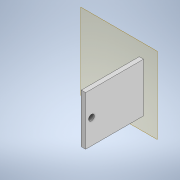
# Autodesk Inventor part: sideSupportFor12inchBase
Saved by Autodesk Inventor 2021 (Build 250183000, 183)
## iProperties
Created: 2020-07-01
Part Number: sideSupportFor12inchBase
Material: Generic
Document SubType Name: Modeling
Designer: robst
Density: 1 g/cm^3
Appearance: Default
Author: robst
Autodesk Inventor part; units mm, degrees
ref_plane "YZ Plane" through (0, 0, 0) normal (1, 0, 0) x (0, 1, 0)
ref_plane "XZ Plane" through (0, 0, 0) normal (0, 1, 0) x (-1, 0, 0)
ref_plane "XY Plane" through (0, 0, 0) normal (0, 0, 1) x (1, 0, 0)
ref_plane "Work Plane1" through (0, 0, 0) normal (0, 0, 1) x (1, 0, 0)
sketch "Sketch1" plane through (0, 0, 0) normal (0, 0, 1) x (1, 0, 0)
  circle A0 centre (0, 0) radius 152.4 projected
  line L0 (107.95, -107.5758) -> (107.95, 107.5758)
  line L1 (88.9, 107.5758) -> (88.9, -107.5758)
  line L2 (88.9, -107.5758) -> (107.95, -107.5758)
  line L3 (88.9, 107.5758) -> (107.95, 107.5758)
  dimension "d0" = 19.05
  dimension "d1" = 88.9
  constraints: 8 end point, 2 point on circle, 2 vertical, 1 perpendicular
  measures "d0" distance of L1.end L0.start
  measures "d1" distance from line of L1 point (0, 0)
extrude "Extrusion1" add sketch "Sketch1" along normal blind 254 contours L0 L2 L1 L3
sketch "Sketch2" plane through (107.95, -107.5758, 0) normal (1, 0, 0) x (0, 0, -1)
  line L0 (-254, 0) -> (-254, 215.1516) construction
  line L1 (-254, 107.5758) -> (0, 107.5758) construction
  circle A0 centre (-228.6, 107.5758) radius 12.7
  dimension "d4" = 25.4
  dimension "d5" = 25.4
  constraints: 2 end point, 1 centre point, 1 horizontal, 1 midpoint, 1 point on line
  measures "d4" diameter of A0
  measures "d5" distance from line of A0.centre L0
extrude "Extrusion2" cut sketch "Sketch2" against normal through all
body "Solid1"
